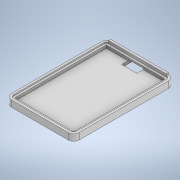
# Autodesk Inventor part: piholder-proto-v3
Saved by Autodesk Inventor 2022 (Build 260153000, 153)
## iProperties
Created: 2021-07-08
Part Number: piholder-proto-v3
Material: Generic
Document SubType Name: Modeling
Designer: dncob
Density: 1 g/cm^3
Appearance: Default
Author: dncob
Autodesk Inventor part; units mm, degrees
ref_plane "YZ Plane" through (0, 0, 0) normal (1, 0, 0) x (0, 1, 0)
ref_plane "XZ Plane" through (0, 0, 0) normal (0, 1, 0) x (-1, 0, 0)
ref_plane "XY Plane" through (0, 0, 0) normal (0, 0, 1) x (1, 0, 0)
sketch "Sketch1" plane through (0, 0, 0) normal (0, 1, 0) x (-1, 0, 0)
  line L0 (-26, 44) -> (26, 44)
  line L1 (29, 41) -> (29, -42)
  line L2 (27, -44) -> (-26, -44)
  line L3 (-29, -41) -> (-29, 41)
  line L4 (-29, 44) -> (29, -44) construction
  line L5 (29, 44) -> (-29, -44) construction
  arc A0 (27, -44) -> (29, -42) centre (27, -42) ccw
  arc A1 (-29, -41) -> (-26, -44) centre (-26, -41) ccw
  arc A2 (-26, 44) -> (-29, 41) centre (-26, 41) ccw
  arc A3 (29, 41) -> (26, 44) centre (26, 41) ccw
  line L6 (31, -42) -> (31, 41)
  arc A4 (31, 41) -> (26, 46) centre (26, 41) ccw
  line L7 (26, 46) -> (-26, 46)
  arc A5 (-26, 46) -> (-31, 41) centre (-26, 41) ccw
  line L8 (-31, 41) -> (-31, -41)
  arc A6 (-31, -41) -> (-26, -46) centre (-26, -41) ccw
  line L9 (-26, -46) -> (27, -46)
  arc A7 (27, -46) -> (31, -42) centre (27, -42) ccw
  point P0 (0, 0)
  dimension "d0" = 58
  dimension "d1" = 88
  dimension "d2" = 2
  dimension "d3" = 3
  dimension "d4" = 2
  constraints: 20 end point, 16 point on circle, 8 centre point, 8 point on line, 8 tangent, 4 parallel, 2 equal radius, 2 midpoint, 2 perpendicular, 1 horizontal, 7 other
  measures "d0" distance of L4.end L5.end
  measures "d1" distance of L5.start L4.end
  measures "d2" radius of A0
  measures "d3" radius of A1
  measures "d4" distance between parallel lines of L1 L6
extrude "Extrusion1" add sketch "Sketch1" along normal blind 1
sketch "Sketch2" plane through (0, 0, 0) normal (0, -1, 0) x (1, 0, 0)
  arc A0 (-26, 46) -> (-31, 41) centre (-26, 41) ccw projected
  line L0 (-26, 46) -> (26, 46) projected
  arc A1 (31, 41) -> (26, 46) centre (26, 41) ccw projected
  line L1 (31, 41) -> (31, -41) projected
  arc A2 (26, -46) -> (31, -41) centre (26, -41) ccw projected
  line L2 (26, -46) -> (-27, -46) projected
  arc A3 (-31, -42) -> (-27, -46) centre (-27, -42) ccw projected
  line L3 (-31, -42) -> (-31, 41) projected
  line L4 (-27, -46) -> (26, -46)
  line L5 (31, -41) -> (31, 41)
  line L6 (26, 46) -> (-26, 46)
  line L7 (-31, 41) -> (-31, -42)
  line L8 (-30, -44.5) -> (30, 44.5) construction
  line L9 (30, -44.5) -> (-30, 44.5) construction
  arc A4 (-26, 46) -> (-31, 41) centre (-26, 41) ccw
  arc A5 (31, 41) -> (26, 46) centre (26, 41) ccw
  arc A6 (26, -44) -> (29, -41) centre (26, -41) ccw projected
  arc A7 (26, -46) -> (31, -41) centre (26, -41) ccw
  arc A8 (-31, -42) -> (-27, -46) centre (-27, -42) ccw
  line L10 (26, 42) -> (-26, 42)
  arc A9 (-26, 42) -> (-27, 41) centre (-26, 41) ccw
  line L11 (-27, 41) -> (-27, -42)
  line L12 (-27, -42) -> (26, -42)
  arc A10 (26, -42) -> (27, -41) centre (26, -41) ccw
  line L13 (27, -41) -> (27, 41)
  arc A11 (27, 41) -> (26, 42) centre (26, 41) ccw
  point P0 (0, 0)
  dimension "d12" = 4
  constraints: 21 end point, 14 point on circle, 7 centre point, 4 coincident, 4 concentric, 4 point on line, 2 collinear, 2 midpoint, 2 parallel, 1 horizontal, 1 perpendicular, 11 other
  measures "d12" distance between parallel lines of L10 L0
extrude "Extrusion2" add sketch "Sketch2" along normal blind 2.5
sketch "Sketch3" plane through (26, 1, -46) normal (0, 0, -1) x (-1, 0, 0)
  line L0 (53, -3.5) -> (53, 0) projected
  line L1 (53, 0) -> (0, 0)
  line L2 (0, 0) -> (0, 1.5)
  line L3 (0, 1.5) -> (53, 1.5)
  line L4 (53, 1.5) -> (53, 0)
  point P0 (26, -1)
  dimension "d9" = 1.5
  constraints: 8 end point, 2 parallel, 1 coincident, 1 horizontal, 1 perpendicular
  measures "d9" distance between parallel lines of L1 L3
extrude "Extrusion3" add sketch "Sketch3" against normal blind 2
sketch "Sketch4" plane through (0, -2.5, 0) normal (0, -1, 0) x (1, 0, 0)
  line L0 (26, 46) -> (-26, 46)
  line L1 (-31, 41) -> (-31, -42)
  line L2 (-27, -46) -> (26, -46)
  line L3 (31, -41) -> (31, 41)
  line L4 (30, 44.5) -> (-30, -44.5) construction
  line L5 (-30, 44.5) -> (30, -44.5) construction
  line L6 (-27, -46) -> (26, -46) projected
  line L7 (-31, 41) -> (-31, -42) projected
  arc A0 (26, -46) -> (31, -41) centre (26, -41) ccw projected
  arc A1 (-31, -42) -> (-27, -46) centre (-27, -42) ccw projected
  arc A2 (-26, 46) -> (-31, 41) centre (-26, 41) ccw projected
  arc A3 (31, 41) -> (26, 46) centre (26, 41) ccw projected
  arc A4 (26, -46) -> (31, -41) centre (26, -41) ccw
  line L8 (26, -42) -> (-27, -42) projected
  arc A5 (-31, -42) -> (-27, -46) centre (-27, -42) ccw
  arc A6 (-26, 46) -> (-31, 41) centre (-26, 41) ccw
  arc A7 (31, 41) -> (26, 46) centre (26, 41) ccw
  line L9 (26, 46) -> (-26, 46) projected
  point P0 (0, 0)
  point P1 (-31, 41)
  point P2 (-31, -42)
  point P3 (26, -46)
  constraints: 13 end point, 10 point on circle, 4 centre point, 4 coincident, 4 concentric, 4 point on line, 3 collinear, 2 midpoint, 2 parallel, 1 horizontal, 1 perpendicular
extrude "Extrusion4" add sketch "Sketch4" along normal blind 2.5
sketch "Sketch5" plane through (26, 2.5, -46) normal (0, 0, -1) x (-1, 0, 0)
  line L0 (53, -7.5) -> (0, -7.5) projected
  line L1 (19, -7.5) -> (33, -7.5)
  line L2 (33, -7.5) -> (33, -4)
  line L3 (33, -4) -> (19, -4)
  line L4 (19, -4) -> (19, -7.5)
  line L5 (19, -7.5) -> (33, -4) construction
  line L6 (33, -7.5) -> (19, -4) construction
  point P0 (26, -2.5)
  point P1 (26, -5.75)
  dimension "d16" = 14
  dimension "d17" = 0
  dimension "d18" = 3.5
  constraints: 12 end point, 2 midpoint, 2 parallel, 1 horizontal, 1 perpendicular, 1 vertical alignment
  measures "d16" distance of L2.end L3.end
  measures "d17" distance between parallel lines of L0 L1
  measures "d18" distance between parallel lines of L1 L3
extrude "Extrusion5" cut sketch "Sketch5" against normal blind 10
body "Solid1"
